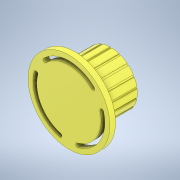
# Autodesk Inventor part: 3inPvcCap
Saved by Autodesk Inventor 2022.2 (Build 262287000, 287)
## iProperties
Created: 2021-11-22
Part Number: 3inPvcCap
Material: PC/ABS Plastic
Document SubType Name: Modeling
Designer: robst
Density: 0.357273 g/cm^3
Appearance: Smooth - Yellow
Author: robst
Autodesk Inventor part; units mm, degrees
ref_plane "YZ Plane" through (0, 0, 0) normal (1, 0, 0) x (0, 1, 0)
ref_plane "XZ Plane" through (0, 0, 0) normal (0, 1, 0) x (-1, 0, 0)
ref_plane "XY Plane" through (0, 0, 0) normal (0, 0, 1) x (1, 0, 0)
sketch "Sketch1" plane through (0, 0, 0) normal (0, 0, 1) x (1, 0, 0)
  circle A0 centre (0, 0) radius 44.45
  circle A1 centre (0, 0) radius 36.83
  circle A2 centre (0, 0) radius 57.15
  circle A3 centre (0, 0) radius 30.48
  dimension "d0" = 88.9
  dimension "d1" = 73.66
  dimension "d4" = 12.7
  dimension "d7" = 6.35
  constraints: 4 centre point, 4 coincident
  measures "d0" diameter of A0
  measures "d1" diameter of A1
  measures "d4" radial gap between concentric circles of A0 A2
  measures "d7" radial gap between concentric circles of A3 A1
extrude "Extrusion2" add sketch "Sketch1" along normal blind 8 contours A0 | A1 | A2 | A3
extrude "Extrusion3" add sketch "Sketch1" against normal blind 50.8 contours A1
sketch "Sketch6" plane through (0, 0, 8) normal (0, 0, 1) x (1, 0, 0)
  arc A0 (33.676, 33.676) -> (-33.676, 33.676) centre (0, 0) ccw construction
  arc A1 (35.481, 35.481) -> (-35.481, 35.481) centre (0, 0) ccw
  arc A2 (31.8709, 31.8709) -> (-31.8709, 31.8709) centre (0, 0) ccw
  arc A3 (31.8709, 31.8709) -> (35.481, 35.481) centre (33.676, 33.676) ccw
  arc A4 (-35.481, 35.481) -> (-31.8709, 31.8709) centre (-33.676, 33.676) ccw
  line L0 (0, 0) -> (33.676, 33.676) construction
  line L1 (0, 0) -> (47.625, 0) construction
  line L2 (0, 0) -> (-33.676, 33.676) construction
  dimension "d26" = 47.625
  dimension "d27" = 45
  dimension "d28" = 90
  dimension "d29" = 5.1054
  constraints: 10 point on circle, 6 end point, 5 centre point, 4 tangent, 1 coincident, 1 equal length, 1 horizontal
  measures "d26" radius of A0
  measures "d27" angle of L1 L0
  measures "d28" angle of L0 L2
  measures "d29" diameter of A4
extrude "Extrusion7" cut sketch "Sketch6" against normal through all
pattern_circular "Circular Pattern1" count 3 over 360 about axis through (0, 0, -10) along (0, 0, 1) of "Extrusion7"
sketch "Sketch8" plane through (0, 0, -50.8) normal (0, 0, -1) x (-1, 0, 0)
  circle A0 centre (0, 0) radius 36.83 projected
  arc A1 (0, 36.83) -> (-1.27, 36.8081) centre (0, 0) ccw
  line L0 (0, 0) -> (0, 36.83) construction
  line L1 (0, 36.83) -> (0, 35.56)
  line L2 (0, 35.56) -> (-1.27, 35.56)
  line L3 (-1.27, 35.56) -> (-1.27, 36.8081)
  circle A2 centre (0, 0) radius 36.83 projected
  circle A3 centre (0, 0) radius 36.83
  line L4 (0, 35.56) -> (1.27, 35.56)
  line L5 (1.27, 35.56) -> (1.27, 36.8081)
  point P0 (-1.27, 36.8081)
  dimension "d35" = 1.27
  dimension "d36" = 1.27
  constraints: 12 end point, 3 point on circle, 2 centre point, 2 symmetric about line, 1 coincident, 1 concentric, 1 horizontal, 1 perpendicular, 1 point on line, 1 vertical, 1 other
  measures "d35" distance of L1.end L0.end
  measures "d36" distance of L1.end L2.end
extrude "Extrusion9" cut sketch "Sketch8" against normal up to surface (50.8 mm away) contours L5 L4 L1 A0 | A0 L1 L2 L3
sketch "Sketch3" plane through (0, 0, 8) normal (0, 0, 1) x (1, 0, 0)
  ellipse E0 centre (0, 0) end of major axis (57.15, 0) minor radius 60.8178
  circle A0 centre (0, 0) radius 57.15 projected
  circle A1 centre (0, 0) radius 57.15
  point P0 (-57.15, 0)
  point P1 (57.15, 0)
  dimension "d11" = 60.8178
  dimension "d12" = 57.15
  constraints: 2 coincident, 1 centre point, 1 concentric, 2 other
pattern_circular "Circular Pattern2" count 18 over 360 about axis through (0, 0, -10) along (0, 0, 1) of "Extrusion9"
equation "\"d0\" = outsideDiameter"
equation "\"d1\" = insideDiameter"
equation "\"d26\" = 0.5 * slotDiameter"
equation "\"d28\" = totalAngleForSlot"
equation "\"d29\" = widthOfSlot"
equation "\"d11\" = 0.5 * elipseMajorDiameter"
equation "\"d12\" = 0.5 * elipseMinorDiameter"
equation "\"insideDiameter\" = 73.66"
equation "\"outsideDiameter\" = 88.9"
equation "\"elipseMajorDiameter\" = 121.63552"
equation "\"elipseMinorDiameter\" = 114.3"
equation "\"widthOfSlot\" = 5.1054"
equation "\"totalAngleForSlot\" = 90deg"
equation "\"slotDiameter\" = 95.25"
body "Solid2"
